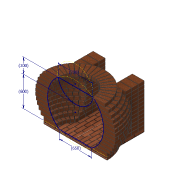
# Autodesk Inventor part: Geometria
Saved by Autodesk Inventor 2019.1 (Build 231200000, 200)
## iProperties
Created: 2019-11-21
Part Number: Geometria
Material: Brick, Common, Brown
Document SubType Name: Modeling
Designer: jjespitia
Density: 1.95 g/cm^3
Appearance: Uniform Running - Orange
Author: jjespitia
Autodesk Inventor part; units mm, degrees
ref_plane "YZ Plane" through (0, 0, 0) normal (1, 0, 0) x (0, 1, 0)
ref_plane "XZ Plane" through (0, 0, 0) normal (0, 1, 0) x (-1, 0, 0)
ref_plane "XY Plane" through (0, 0, 0) normal (0, 0, 1) x (1, 0, 0)
sketch "Sketch1" plane through (0, 0, 0) normal (0, 0, 1) x (1, 0, 0)
  circle A0 centre (0, 494.7917) radius 354.1667
  circle A1 centre (0, 0) radius 562.717
  line L0 (-325, -459.375) -> (325, -459.375)
  line L1 (-350, 440.625) -> (350, 440.625)
  line L2 (-350, 440.625) -> (0, 0)
  line L3 (0, 0) -> (0, 440.625)
  line L4 (0, -459.375) -> (0, 0)
  line L5 (0, 0) -> (-325, -459.375)
  dimension "d0" = 300
  dimension "d1" = 700
  dimension "d4" = 650
  dimension "d6" = 600
  dimension "d7" = 562.717
  dimension "d8" = 440.625
  dimension "d9" = 459.375
  constraints: 12 end point, 6 point on circle, 2 centre point, 2 horizontal, 2 midpoint, 1 coincident, 1 vertical
  measures "d0" distance edge to line of A0 L1
  measures "d1" distance of L1.start L1.end
  measures "d4" distance of L0.start L0.end
  measures "d6" distance edge to line of A0 L0
  measures "d7" distance of L1.start L2.end
  measures "d8" distance of L2.end L3.end
  measures "d9" distance of L4.start L2.end
sketch "Sketch2" plane through (0, 0, 0) normal (0, 0, 1) x (1, 0, 0)
  arc A0 (325, -459.375) -> (350, 440.625) centre (0, 0) ccw construction
  line L0 (562.3389, 20.625) -> (802.3389, 20.625)
  line L1 (802.3389, 20.625) -> (802.3389, -39.375)
  line L2 (802.3389, -39.375) -> (562.3389, -39.375)
  line L3 (562.3389, -39.375) -> (562.3389, 20.625)
  line L4 (560.5466, -49.375) -> (800.5466, -49.375)
  line L5 (800.5466, -49.375) -> (800.5466, -109.375)
  line L6 (800.5466, -109.375) -> (560.5466, -109.375)
  line L7 (560.5466, -109.375) -> (560.5466, -49.375)
  line L8 (549.9091, -119.375) -> (789.9091, -119.375)
  line L9 (789.9091, -119.375) -> (789.9091, -179.375)
  line L10 (789.9091, -179.375) -> (549.9091, -179.375)
  line L11 (549.9091, -179.375) -> (549.9091, -119.375)
  line L12 (350, 440.625) -> (590, 440.625)
  line L13 (590, 440.625) -> (590, 380.625)
  line L14 (590, 380.625) -> (350, 380.625)
  line L15 (350, 380.625) -> (350, 440.625)
  line L16 (423.4235, 370.625) -> (663.4235, 370.625)
  line L17 (663.4235, 370.625) -> (663.4235, 310.625)
  line L18 (663.4235, 310.625) -> (423.4235, 310.625)
  line L19 (423.4235, 310.625) -> (423.4235, 370.625)
  line L20 (475.6837, 300.625) -> (715.6837, 300.625)
  line L21 (715.6837, 300.625) -> (715.6837, 240.625)
  line L22 (715.6837, 240.625) -> (475.6837, 240.625)
  line L23 (475.6837, 240.625) -> (475.6837, 300.625)
  line L24 (513.286, 230.625) -> (753.286, 230.625)
  line L25 (753.286, 230.625) -> (753.286, 170.625)
  line L26 (753.286, 170.625) -> (513.286, 170.625)
  line L27 (513.286, 170.625) -> (513.286, 230.625)
  line L28 (539.3051, 160.625) -> (779.3051, 160.625)
  line L29 (779.3051, 160.625) -> (779.3051, 100.625)
  line L30 (779.3051, 100.625) -> (539.3051, 100.625)
  line L31 (539.3051, 100.625) -> (539.3051, 160.625)
  line L32 (555.3715, 90.625) -> (795.3715, 90.625)
  line L33 (795.3715, 90.625) -> (795.3715, 30.625)
  line L34 (795.3715, 30.625) -> (555.3715, 30.625)
  line L35 (555.3715, 30.625) -> (555.3715, 90.625)
  line L36 (529.8939, -189.375) -> (769.8939, -189.375)
  line L37 (769.8939, -189.375) -> (769.8939, -249.375)
  line L38 (769.8939, -249.375) -> (529.8939, -249.375)
  line L39 (529.8939, -249.375) -> (529.8939, -189.375)
  line L40 (499.3746, -259.375) -> (739.3746, -259.375)
  line L41 (739.3746, -259.375) -> (739.3746, -319.375)
  line L42 (739.3746, -319.375) -> (499.3746, -319.375)
  line L43 (499.3746, -319.375) -> (499.3746, -259.375)
  line L44 (456.2483, -329.375) -> (696.2483, -329.375)
  line L45 (696.2483, -329.375) -> (696.2483, -389.375)
  line L46 (696.2483, -389.375) -> (456.2483, -389.375)
  line L47 (456.2483, -389.375) -> (456.2483, -329.375)
  line L48 (396.4215, -399.375) -> (636.4215, -399.375)
  line L49 (636.4215, -399.375) -> (636.4215, -459.375)
  line L50 (636.4215, -459.375) -> (396.4215, -459.375)
  line L51 (396.4215, -459.375) -> (396.4215, -399.375)
  line L52 (0, -459.375) -> (636.4215, -459.375)
  line L53 (636.4215, -459.375) -> (636.4215, -519.375)
  line L54 (636.4215, -519.375) -> (0, -519.375)
  line L55 (0, -519.375) -> (0, -459.375)
  line L56 (0, -845.052) -> (0, 1131.2934) projected
  point P0 (0, 440.625)
  dimension "d10" = 60
  dimension "d11" = 240
  dimension "d15" = 60
  dimension "d16" = 240
  dimension "d17" = 60
  dimension "d18" = 240
  dimension "d19" = 10
  dimension "d20" = 10
  dimension "d21" = 60
  dimension "d22" = 240
  dimension "d23" = 60
  dimension "d24" = 240
  dimension "d25" = 60
  dimension "d26" = 240
  dimension "d27" = 10
  dimension "d28" = 10
  dimension "d29" = 60
  dimension "d30" = 240
  dimension "d31" = 60
  dimension "d32" = 240
  dimension "d33" = 60
  dimension "d34" = 240
  dimension "d35" = 10
  dimension "d36" = 10
  dimension "d37" = 10
  dimension "d38" = 10
  dimension "d39" = 60
  dimension "d40" = 240
  dimension "d41" = 60
  dimension "d42" = 240
  dimension "d43" = 60
  dimension "d44" = 240
  dimension "d45" = 10
  dimension "d46" = 10
  dimension "d47" = 60
  dimension "d48" = 240
  dimension "d55" = 10
  dimension "d56" = 10
  constraints: 112 end point, 28 parallel, 14 horizontal, 14 perpendicular, 2 coincident, 1 collinear, 1 point on line, 16 other
  measures "d10" distance of L0.end L1.end
  measures "d11" distance of L0.start L0.end
  measures "d15" distance of L4.end L5.end
  measures "d16" distance of L4.start L4.end
  measures "d17" distance of L8.end L9.end
  measures "d18" distance of L8.start L8.end
  measures "d19" distance between parallel lines of L4 L2
  measures "d20" distance between parallel lines of L8 L6
  measures "d21" distance of L13.start L13.end
  measures "d22" distance of L12.start L13.start
  measures "d23" distance of L16.end L18.start
  measures "d24" distance of L16.start L16.end
  measures "d25" distance of L20.end L21.end
  measures "d26" distance of L23.end L20.end
  measures "d27" distance between parallel lines of L16 L14
  measures "d28" distance between parallel lines of L20 L18
  measures "d29" distance of L25.start L25.end
  measures "d30" distance of L24.start L25.start
  measures "d31" distance of L28.end L30.start
  measures "d32" distance of L28.start L28.end
  measures "d33" distance of L32.end L33.end
  measures "d34" distance of L35.end L32.end
  measures "d35" distance between parallel lines of L28 L26
  measures "d36" distance between parallel lines of L32 L30
  measures "d37" distance between parallel lines of L22 L24
  measures "d38" distance between parallel lines of L34 L0
  measures "d39" distance of L37.start L37.end
  measures "d40" distance of L36.start L37.start
  measures "d41" distance of L40.end L42.start
  measures "d42" distance of L40.start L40.end
  measures "d43" distance of L44.end L45.end
  measures "d44" distance of L47.end L44.end
  measures "d45" distance between parallel lines of L40 L38
  measures "d46" distance between parallel lines of L44 L42
  measures "d47" distance of L49.start L49.end
  measures "d48" distance of L48.start L49.start
  measures "d55" distance between parallel lines of L10 L36
  measures "d56" distance between parallel lines of L48 L46
revolve "Revolution1" add sketch "Sketch2" angle 180 about axis through (0, -10, 0) along (0, 1, 0) contours L0 L1 L2 L3 | L8 L9 L10 L11 | L12 L13 L14 L15 | L20 L21 L22 L23 | L28 L29 L30 L31 | L40 L41 L42 L43 | L48 L49 L50 L51
revolve "Revolution2" add sketch "Sketch2" angle 180 about axis through (0, -10, 0) along (0, 1, 0) separate body contours L4 L5 L6 L7 | L16 L17 L18 L19 | L24 L25 L26 L27 | L32 L33 L34 L35 | L36 L37 L38 L39 | L44 L45 L46 L47 | L50 L53 L54 L55 L52
sketch "Sketch3" plane through (350, 440.625, 0) normal (0, 0, 1) x (1, 0, 0)
  line L0 (-625, -70) -> (-75, -70)
  line L1 (-75, -70) -> (-75, -900)
  line L2 (-75, -900) -> (-625, -900)
  line L3 (-625, -900) -> (-625, -70)
  line L4 (73.4235, -70) -> (-773.4235, -70) projected
  line L5 (286.4215, -900) -> (-986.4215, -900) projected
  point P0 (-350, -440.625)
  point P1 (-350, -70)
  dimension "d60" = 550
  constraints: 8 end point, 2 parallel, 2 point on line, 1 horizontal, 1 midpoint, 1 perpendicular, 1 vertical alignment
  measures "d60" distance of L1.end L2.end
extrude "Extrusion1" cut sketch "Sketch3" against normal through all bodies 2 1
sketch "Sketch4" plane through (0, -459.375, 0) normal (0, 1, 0) x (1, 0, 0)
  line L0 (275, 490.5099) -> (-275, 490.5099) construction
  line L1 (515, 490.5099) -> (275, 490.5099)
  line L2 (275, 490.5099) -> (275, 610.5099)
  line L3 (275, 610.5099) -> (515, 610.5099)
  line L4 (515, 610.5099) -> (515, 490.5099)
  line L5 (-275, 490.5099) -> (-515, 490.5099)
  line L6 (-515, 490.5099) -> (-515, 610.5099)
  line L7 (-515, 610.5099) -> (-275, 610.5099)
  line L8 (-275, 610.5099) -> (-275, 490.5099)
  line L9 (515, 620.5099) -> (275, 620.5099)
  line L10 (275, 620.5099) -> (275, 740.5099)
  line L11 (275, 740.5099) -> (515, 740.5099)
  line L12 (515, 740.5099) -> (515, 620.5099)
  line L13 (-275, 620.5099) -> (-515, 620.5099)
  line L14 (-515, 620.5099) -> (-515, 740.5099)
  line L15 (-515, 740.5099) -> (-275, 740.5099)
  line L16 (-275, 740.5099) -> (-275, 620.5099)
  line L17 (515, 870.5099) -> (275, 870.5099)
  line L18 (275, 870.5099) -> (275, 750.5099)
  line L19 (275, 750.5099) -> (515, 750.5099)
  line L20 (515, 750.5099) -> (515, 870.5099)
  line L21 (-275, 870.5099) -> (-515, 870.5099)
  line L22 (-515, 870.5099) -> (-515, 750.5099)
  line L23 (-515, 750.5099) -> (-275, 750.5099)
  line L24 (-275, 750.5099) -> (-275, 870.5099)
  point P0 (0, 0)
  point P1 (-275, 490.5099)
  dimension "d63" = 120
  dimension "d64" = 240
  dimension "d65" = 10
  dimension "d66" = 10
  dimension "d67" = 10
  dimension "d68" = 10
  constraints: 51 end point, 12 parallel, 10 equal length, 7 horizontal, 6 perpendicular, 4 collinear, 1 coincident
  measures "d63" distance between parallel lines of L3 L1
  measures "d64" distance between parallel lines of L4 L2
  measures "d65" distance between parallel lines of L3 L9
  measures "d66" distance between parallel lines of L7 L13
  measures "d67" distance between parallel lines of L19 L11
  measures "d68" distance between parallel lines of L23 L15
extrude "Extrusion2" add sketch "Sketch4" along normal up to surface (830 mm away) separate body
sketch "Sketch5" plane through (636.4215, -519.375, 0) normal (0, 0, 1) x (1, 0, 0)
  line L0 (-1438.7604, 830) -> (165.9174, 830)
  line L1 (165.9174, 830) -> (165.9174, 820)
  line L2 (165.9174, 820) -> (-1438.7604, 820)
  line L3 (-1438.7604, 820) -> (-1438.7604, 830)
  line L4 (-1438.7604, 540) -> (-1438.7604, 480) projected
  line L5 (165.9174, 540) -> (165.9174, 480) projected
  line L6 (-1438.7604, 760) -> (165.9174, 760)
  line L7 (165.9174, 760) -> (165.9174, 750)
  line L8 (165.9174, 750) -> (-1438.7604, 750)
  line L9 (-1438.7604, 750) -> (-1438.7604, 760)
  line L10 (-1438.7604, 690) -> (165.9174, 690)
  line L11 (165.9174, 690) -> (165.9174, 680)
  line L12 (165.9174, 680) -> (-1438.7604, 680)
  line L13 (-1438.7604, 680) -> (-1438.7604, 690)
  line L14 (-1438.7604, 620) -> (165.9174, 620)
  line L15 (165.9174, 620) -> (165.9174, 610)
  line L16 (165.9174, 610) -> (-1438.7604, 610)
  line L17 (-1438.7604, 610) -> (-1438.7604, 620)
  line L18 (-1438.7604, 550) -> (165.9174, 550)
  line L19 (165.9174, 550) -> (165.9174, 540)
  line L20 (165.9174, 540) -> (-1438.7604, 540)
  line L21 (-1438.7604, 540) -> (-1438.7604, 550)
  line L22 (-1438.7604, 480) -> (165.9174, 480)
  line L23 (165.9174, 480) -> (165.9174, 470)
  line L24 (165.9174, 470) -> (-1438.7604, 470)
  line L25 (-1438.7604, 470) -> (-1438.7604, 480)
  line L26 (-1438.7604, 410) -> (165.9174, 410)
  line L27 (165.9174, 410) -> (165.9174, 400)
  line L28 (165.9174, 400) -> (-1438.7604, 400)
  line L29 (-1438.7604, 400) -> (-1438.7604, 410)
  line L30 (-1438.7604, 340) -> (165.9174, 340)
  line L31 (165.9174, 340) -> (165.9174, 330)
  line L32 (165.9174, 330) -> (-1438.7604, 330)
  line L33 (-1438.7604, 330) -> (-1438.7604, 340)
  line L34 (-1438.7604, 270) -> (165.9174, 270)
  line L35 (165.9174, 270) -> (165.9174, 260)
  line L36 (165.9174, 260) -> (-1438.7604, 260)
  line L37 (-1438.7604, 260) -> (-1438.7604, 270)
  line L38 (-1438.7604, 200) -> (165.9174, 200)
  line L39 (165.9174, 200) -> (165.9174, 190)
  line L40 (165.9174, 190) -> (-1438.7604, 190)
  line L41 (-1438.7604, 190) -> (-1438.7604, 200)
  line L42 (-1438.7604, 130) -> (165.9174, 130)
  line L43 (165.9174, 130) -> (165.9174, 120)
  line L44 (165.9174, 120) -> (-1438.7604, 120)
  line L45 (-1438.7604, 120) -> (-1438.7604, 130)
  point P0 (-636.4215, 519.375)
  point P1 (27.0021, 830)
  point P2 (79.2622, 820)
  point P3 (27.0021, 760)
  point P4 (79.2622, 750)
  point P5 (27.0021, 690)
  point P6 (79.2622, 680)
  point P7 (27.0021, 620)
  point P8 (79.2622, 610)
  point P9 (27.0021, 550)
  point P10 (79.2622, 540)
  point P11 (27.0021, 480)
  point P12 (79.2622, 470)
  point P13 (27.0021, 410)
  point P14 (79.2622, 400)
  point P15 (27.0021, 340)
  point P16 (79.2622, 330)
  point P17 (27.0021, 270)
  point P18 (79.2622, 260)
  point P19 (27.0021, 200)
  point P20 (79.2622, 190)
  point P21 (27.0021, 130)
  point P22 (79.2622, 120)
  dimension "d73" = 70
  constraints: 88 end point, 22 point on line, 3 collinear, 2 parallel, 1 horizontal, 1 perpendicular, 1 vertical, 99 other
  measures "d73" distance of L0.start L6.start
extrude "Extrusion3" cut sketch "Sketch5" against normal up to surface (870.5099 mm away) contours L0 L1 L2 L3 | L21 L18 L19 L20 | L22 L23 L24 L25 | L6 L7 L8 L9 | L10 L11 L12 L13 | L14 L15 L16 L17 | L26 L27 L28 L29 | L30 L31 L32 L33 | L34 L35 L36 L37 | L38 L39 L40 L41 | L42 L43 L44 L45 bodies 3
sketch "Sketch6" plane through (350, 440.625, 0) normal (0, 1, 0) x (1, 0, 0)
  arc A0 (0, 0) -> (-700, 0) centre (-350, 0) ccw projected
  line L0 (-350.7786, 4.939) -> (-349.2214, -4.939)
  line L1 (-349.2214, -4.939) -> (572.3389, 140.34)
  line L2 (572.3389, 140.34) -> (570.7817, 150.218)
  line L3 (570.7817, 150.218) -> (-350.7786, 4.939)
  arc A1 (452.3389, 0) -> (-75, 753.7391) centre (-350, 0) ccw construction
  line L4 (-351.5026, 4.7689) -> (-348.4974, -4.7689)
  line L5 (-348.4974, -4.7689) -> (541.3175, 275.6038)
  line L6 (541.3175, 275.6038) -> (538.3122, 285.1415)
  line L7 (538.3122, 285.1415) -> (-351.5026, 4.7689)
  line L8 (-352.1934, 4.4932) -> (-347.8066, -4.4932)
  line L9 (-347.8066, -4.4932) -> (490.5748, 404.7695)
  line L10 (490.5748, 404.7695) -> (486.188, 413.756)
  line L11 (486.188, 413.756) -> (-352.1934, 4.4932)
  line L12 (-352.8356, 4.1181) -> (-347.1644, -4.1181)
  line L13 (-347.1644, -4.1181) -> (421.2334, 524.9793)
  line L14 (421.2334, 524.9793) -> (415.5621, 533.2156)
  line L15 (415.5621, 533.2156) -> (-352.8356, 4.1181)
  line L16 (-353.4151, 3.652) -> (-346.5849, -3.652)
  line L17 (-346.5849, -3.652) -> (334.8278, 633.5734)
  line L18 (334.8278, 633.5734) -> (327.9975, 640.8773)
  line L19 (327.9975, 640.8773) -> (-353.4151, 3.652)
  line L20 (-353.9191, 3.105) -> (-346.0809, -3.105)
  line L21 (-346.0809, -3.105) -> (233.2695, 728.149)
  line L22 (233.2695, 728.149) -> (225.4314, 734.3589)
  line L23 (225.4314, 734.3589) -> (-353.9191, 3.105)
  line L24 (-354.3363, 2.4893) -> (-345.6637, -2.4893)
  line L25 (-345.6637, -2.4893) -> (118.8059, 806.6135)
  line L26 (118.8059, 806.6135) -> (110.1333, 811.5921)
  line L27 (110.1333, 811.5921) -> (-354.3363, 2.4893)
  line L28 (-354.6576, 1.8185) -> (-345.3424, -1.8185)
  line L29 (-345.3424, -1.8185) -> (-6.0306, 867.2309)
  line L30 (-6.0306, 867.2309) -> (-15.3458, 870.8679)
  line L31 (-15.3458, 870.8679) -> (-354.6576, 1.8185)
  line L32 (-354.8758, 1.1075) -> (-345.1242, -1.1075)
  line L33 (-345.1242, -1.1075) -> (-138.4778, 908.6598)
  line L34 (-138.4778, 908.6598) -> (-148.2294, 910.8748)
  line L35 (-148.2294, 910.8748) -> (-354.8758, 1.1075)
  line L36 (-354.9861, 0.372) -> (-345.0139, -0.372)
  line L37 (-345.0139, -0.372) -> (-275.6051, 929.9837)
  line L38 (-275.6051, 929.9837) -> (-285.5774, 930.7277)
  line L39 (-285.5774, 930.7277) -> (-354.9861, 0.372)
  line L40 (-354.9862, -0.3718) -> (-345.0138, 0.3718)
  line L41 (-345.0138, 0.3718) -> (-414.3785, 930.7307)
  line L42 (-414.3785, 930.7307) -> (-424.3509, 929.9872)
  line L43 (-424.3509, 929.9872) -> (-354.9862, -0.3718)
  line L44 (-354.8759, -1.1073) -> (-345.1241, 1.1073)
  line L45 (-345.1241, 1.1073) -> (-551.7275, 910.8844)
  line L46 (-551.7275, 910.8844) -> (-561.4792, 908.6698)
  line L47 (-561.4792, 908.6698) -> (-354.8759, -1.1073)
  line L48 (-354.6577, -1.8183) -> (-345.3423, 1.8183)
  line L49 (-345.3423, 1.8183) -> (-684.613, 870.8837)
  line L50 (-684.613, 870.8837) -> (-693.9283, 867.2471)
  line L51 (-693.9283, 867.2471) -> (-354.6577, -1.8183)
  line L52 (-354.3364, -2.4891) -> (-345.6636, 2.4891)
  line L53 (-345.6636, 2.4891) -> (-810.0949, 811.6138)
  line L54 (-810.0949, 811.6138) -> (-818.7677, 806.6357)
  line L55 (-818.7677, 806.6357) -> (-354.3364, -2.4891)
  line L56 (-353.9192, -3.1048) -> (-346.0808, 3.1048)
  line L57 (-346.0808, 3.1048) -> (-925.3966, 734.3861)
  line L58 (-925.3966, 734.3861) -> (-933.2351, 728.1766)
  line L59 (-933.2351, 728.1766) -> (-353.9192, -3.1048)
  line L60 (-353.4153, -3.6518) -> (-346.5847, 3.6518)
  line L61 (-346.5847, 3.6518) -> (-1027.9671, 640.9094)
  line L62 (-1027.9671, 640.9094) -> (-1034.7978, 633.6058)
  line L63 (-1034.7978, 633.6058) -> (-353.4153, -3.6518)
  line L64 (-352.8358, -4.118) -> (-347.1642, 4.118)
  line L65 (-347.1642, 4.118) -> (-1115.5369, 533.2518)
  line L66 (-1115.5369, 533.2518) -> (-1121.2086, 525.0158)
  line L67 (-1121.2086, 525.0158) -> (-352.8358, -4.118)
  line L68 (-352.1936, -4.4931) -> (-347.8064, 4.4931)
  line L69 (-347.8064, 4.4931) -> (-1186.1684, 413.7955)
  line L70 (-1186.1684, 413.7955) -> (-1190.5556, 404.8093)
  line L71 (-1190.5556, 404.8093) -> (-352.1936, -4.4931)
  line L72 (-351.5029, -4.7688) -> (-348.4971, 4.7688)
  line L73 (-348.4971, 4.7688) -> (-1238.2987, 285.1836)
  line L74 (-1238.2987, 285.1836) -> (-1241.3044, 275.646)
  line L75 (-1241.3044, 275.646) -> (-351.5029, -4.7688)
  line L76 (-350.7788, -4.939) -> (-349.2212, 4.939)
  line L77 (-349.2212, 4.939) -> (-1270.7745, 150.2616)
  line L78 (-1270.7745, 150.2616) -> (-1272.3322, 140.3837)
  line L79 (-1272.3322, 140.3837) -> (-350.7788, -4.939)
  line L80 (429.3051, 0) -> (189.3051, 0) projected
  point P0 (-350, 0)
  point P1 (-350, 0)
  point P2 (443.3143, 120)
  point P3 (-350, 0)
  point P4 (-3.8721, 51.9177)
  point P5 (-350, 0)
  point P6 (416.7375, 236.3498)
  point P7 (443.4626, 119.016)
  point P8 (-350, 0)
  point P9 (-15.4026, 102.6867)
  point P10 (-350, 0)
  point P11 (373.1958, 347.4701)
  point P12 (417.0301, 235.3986)
  point P13 (-350, 0)
  point P14 (-34.3364, 151.1836)
  point P15 (-350, 0)
  point P16 (313.6527, 450.9022)
  point P17 (373.6262, 346.5728)
  point P18 (-350, 0)
  point P19 (-60.2546, 196.3354)
  point P20 (-350, 0)
  point P21 (239.4255, 544.3576)
  point P22 (314.2114, 450.0787)
  point P23 (-350, 0)
  point P24 (-92.5837, 237.1432)
  point P25 (-350, 0)
  point P26 (152.1566, 625.7686)
  point P27 (240.1002, 543.6262)
  point P28 (-350, 0)
  point P29 (-130.6085, 272.7038)
  point P30 (-350, 0)
  point P31 (53.7771, 693.3338)
  point P32 (152.9324, 625.1453)
  point P33 (-350, 0)
  point P34 (-173.4875, 302.2306)
  point P35 (-350, 0)
  point P36 (-53.5365, 745.5582)
  point P37 (54.6367, 692.8325)
  point P38 (-350, 0)
  point P39 (-220.272, 325.0702)
  point P40 (-350, 0)
  point P41 (-167.4097, 781.2864)
  point P42 (-52.6121, 745.19)
  point P43 (-350, 0)
  point P44 (-269.927, 340.7173)
  point P45 (-350, 0)
  point P46 (-285.3228, 799.7278)
  point P47 (-166.4408, 781.0593)
  point P48 (-350, 0)
  point P49 (-321.3536, 348.8257)
  point P50 (-350, 0)
  point P51 (-404.667, 800.4743)
  point P52 (-284.331, 799.6469)
  point P53 (-350, 0)
  point P54 (-373.414, 349.216)
  point P55 (-350, 0)
  point P56 (-522.8017, 783.5096)
  point P57 (-403.6742, 800.5415)
  point P58 (-350, 0)
  point P59 (-424.9564, 341.8794)
  point P60 (-350, 0)
  point P61 (-637.1129, 749.2088)
  point P62 (-521.8298, 783.7233)
  point P63 (-350, 0)
  point P64 (-474.8403, 326.9784)
  point P65 (-350, 0)
  point P66 (-745.0714, 698.331)
  point P67 (-636.1834, 749.5643)
  point P68 (-350, 0)
  point P69 (-521.9619, 304.8427)
  point P70 (-350, 0)
  point P71 (-844.2886, 632.0019)
  point P72 (-744.205, 698.8205)
  point P73 (-350, 0)
  point P74 (-565.2788, 275.962)
  point P75 (-350, 0)
  point P76 (-932.5691, 551.6891)
  point P77 (-843.5044, 632.6145)
  point P78 (-350, 0)
  point P79 (-603.8323, 240.9754)
  point P80 (-350, 0)
  point P81 (-1007.9597, 459.1696)
  point P82 (-931.8844, 552.4112)
  point P83 (-350, 0)
  point P84 (-636.7696, 200.6569)
  point P85 (-350, 0)
  point P86 (-1068.7922, 356.4905)
  point P87 (-1007.3897, 459.9853)
  point P88 (-350, 0)
  point P89 (-663.3618, 155.8987)
  point P90 (-350, 0)
  point P91 (-1113.7206, 245.9236)
  point P92 (-1068.3495, 357.3817)
  point P93 (-350, 0)
  point P94 (-683.0205, 107.6911)
  point P95 (-350, 0)
  point P96 (-1141.751, 129.9155)
  point P97 (-1113.415, 246.8707)
  dimension "d82" = 10
  dimension "d83" = 120
  dimension "d84" = 120
  dimension "d87" = 162.08
  dimension "d89" = 8.959
  constraints: 160 end point, 21 coincident, 20 point on line, 2 parallel, 1 midpoint, 1 perpendicular, 1 point on circle, 285 other
  measures "d82" distance between parallel lines of L1 L3
  measures "d83" vertical distance of A1.start point (443.314, 120)
  measures "d84" horizontal distance of L1.end A1.start
  measures "d89" angle of L80 L1
extrude "Extrusion4" cut sketch "Sketch6" against normal up to surface (900 mm away) contours L1 L0 L4 L5 L3 A0 | A0 L3 L2 L1 | L5 L3 L9 L7 A0 | A0 L7 L6 L5 | L5 L4 L8 L9 L3 | L4 L7 L77 L3 L0 | L8 L11 L77 L7 L4 | L12 L15 L77 L11 L8 | L12 L13 L3 L9 L8 | L16 L19 L77 L15 L12 | L16 L17 L3 L13 L12 | L20 L23 L77 L19 L16 | L20 L21 L3 L17 L16 | L24 L27 L77 L23 L20 | L24 L25 L3 L21 L20 | L28 L31 L77 L27 L24 | L28 L29 L3 L25 L24 | L32 L35 L77 L31 L28 | L32 L33 L3 L29 L28 | L36 L39 L77 L35 L32 | L36 L37 L3 L33 L32 | L40 L43 L77 L39 L36 | L40 L41 L3 L37 L36 | L44 L47 L77 L43 L40 | L44 L45 L3 L41 L40 | L48 L51 L77 L47 L44 | L48 L49 L3 L45 L44 | L52 L55 L77 L51 L48 | L52 L53 L3 L49 L48 | L56 L59 L77 L55 L52 | L56 L57 L3 L53 L52 | L60 L63 L77 L59 L56 | L60 L61 L3 L57 L56 | L64 L67 L77 L63 L60 | L64 L65 L3 L61 L60 | L68 L71 L77 L67 L64 | L68 L69 L3 L65 L64 | L72 L75 L77 L71 L68 | L72 L73 L3 L69 L68 | L76 L79 A0 L77 L75 L72 | L76 L77 L3 L73 L72 | L0 L3 L77 L76 | L3 L13 L7 L9 | L9 L7 L13 L11 A0 | A0 L11 L10 L9 | L3 L17 L7 L13 | L77 L7 L73 L3 | L77 L11 L73 L7 | L77 L15 L73 L11 | L77 L19 L73 L15 | L77 L23 L73 L19 | L3 L21 L7 L17 | L77 L27 L73 L23 | L3 L25 L7 L21 | L77 L31 L73 L27 | L3 L29 L7 L25 | L77 L35 L73 L31 | L3 L33 L7 L29 | L77 L39 L73 L35 | L3 L37 L7 L33 | L77 L43 L73 L39 | L3 L41 L7 L37 | L77 L47 L73 L43 | L3 L45 L7 L41 | L77 L51 L73 L47 | L3 L49 L7 L45 | L77 L55 L73 L51 | L3 L53 L7 L49 | L77 L59 L73 L55 | L3 L57 L7 L53 | L77 L63 L73 L59 | L3 L61 L7 L57 | L77 L67 L73 L63 | L3 L65 L7 L61 | L77 L71 L73 L67 | L3 L69 L7 L65 | L77 L75 A0 L73 L71 | L3 L73 L7 L69 | L79 L78 L77 A0 | L7 L17 L11 L13 | L73 L11 L69 L7 | L73 L15 L69 L11 | L73 L19 L69 L15 | L73 L23 L69 L19 | L7 L21 L11 L17 | L73 L27 L69 L23 | L7 L25 L11 L21 | L73 L31 L69 L27 | L7 L29 L11 L25 | L73 L35 L69 L31 | L7 L33 L11 L29 | L73 L39 L69 L35 | L7 L37 L11 L33 | L73 L43 L69 L39 | L7 L41 L11 L37 | L73 L47 L69 L43 | L7 L45 L11 L41 | L73 L51 L69 L47 | L7 L49 L11 L45 | L73 L55 L69 L51 | L7 L53 L11 L49 | L73 L59 L69 L55 | L7 L57 L11 L53 | L73 L63 L69 L59 | L7 L61 L11 L57 | L73 L67 L69 L63 | L7 L65 L11 L61 | L73 L71 A0 L69 L67 | L7 L69 L11 L65 | L75 L74 L73 A0 | L13 L11 L17 L15 A0 | A0 L15 L14 L13 | L69 L15 L65 L11 | L69 L19 L65 L15 | L69 L23 L65 L19 | L11 L21 L15 L17 | L69 L27 L65 L23 | L11 L25 L15 L21 | L69 L31 L65 L27 | L11 L29 L15 L25 | L69 L35 L65 L31 | L11 L33 L15 L29 | L69 L39 L65 L35 | L11 L37 L15 L33 | L69 L43 L65 L39 | L11 L41 L15 L37 | L69 L47 L65 L43 | L11 L45 L15 L41 | L69 L51 L65 L47 | L11 L49 L15 L45 | L69 L55 L65 L51 | L11 L53 L15 L49 | L69 L59 L65 L55 | L11 L57 L15 L53 | L69 L63 L65 L59 | L11 L61 L15 L57 | L69 L67 A0 L65 L63 | L11 L65 L15 L61 | L71 L70 L69 A0 | L65 L19 L61 L15 | L65 L23 L61 L19 | L15 L21 L19 A0 L17 | L65 L27 L61 L23 | L15 L25 L19 L21 | L65 L31 L61 L27 | L15 L29 L19 L25 | L65 L35 L61 L31 | L15 L33 L19 L29 | L65 L39 L61 L35 | L15 L37 L19 L33 | L65 L43 L61 L39 | L15 L41 L19 L37 | L65 L47 L61 L43 | L15 L45 L19 L41 | L65 L51 L61 L47 | L15 L49 L19 L45 | L65 L55 L61 L51 | L15 L53 L19 L49 | L65 L59 L61 L55 | L15 L57 L19 L53 | L65 L63 A0 L61 L59 | L15 L61 L19 L57 | L67 L66 L65 A0 | A0 L19 L18 L17 | L61 L23 L57 L19 | L61 L27 L57 L23 | L19 L25 L23 A0 L21 | L61 L31 L57 L27 | L19 L29 L23 L25 | L61 L35 L57 L31 | L19 L33 L23 L29 | L61 L39 L57 L35 | L19 L37 L23 L33 | L61 L43 L57 L39 | L19 L41 L23 L37 | L61 L47 L57 L43 | L19 L45 L23 L41 | L61 L51 L57 L47 | L19 L49 L23 L45 | L61 L55 L57 L51 | L19 L53 L23 L49 | L61 L59 A0 L57 L55 | L19 L57 L23 L53 | L63 L62 L61 A0 | L57 L27 L53 L23 | A0 L23 L22 L21 | L57 L31 L53 L27 | L23 L29 L27 A0 L25 | L57 L35 L53 L31 | L23 L33 L27 L29 | L57 L39 L53 L35 | L23 L37 L27 L33 | L57 L43 L53 L39 | L23 L41 L27 L37 | L57 L47 L53 L43 | L23 L45 L27 L41 | L57 L51 L53 L47 | L23 L49 L27 L45 | L57 L55 A0 L53 L51 | L23 L53 L27 L49 | L59 L58 L57 A0 | L53 L31 L49 L27 | A0 L27 L26 L25 | L53 L35 L49 L31 | L27 L33 L31 A0 L29 | L53 L39 L49 L35 | L27 L37 L31 L33 | L53 L43 L49 L39 | L27 L41 L31 L37 | L53 L47 L49 L43 | L27 L45 L31 L41 | L53 L51 A0 L49 L47 | L27 L49 L31 L45 | L55 L54 L53 A0 | L49 L35 L45 L31 | A0 L31 L30 L29 | L49 L39 L45 L35 | L31 L37 L35 A0 L33 | L49 L43 L45 L39 | L31 L41 L35 L37 | L49 L47 A0 L45 L43 | L31 L45 L35 L41 | L51 L50 L49 A0 | L45 L39 L41 L35 | A0 L35 L34 L33 | L45 L43 A0 L41 L39 | L35 L41 L39 A0 L37 | L47 L46 L45 A0 | A0 L39 L38 L37 | L43 L42 L41 A0 bodies 1
sketch "Sketch7" plane through (-663.4235, 370.625, 0) normal (0, 1, 0) x (1, 0, 0)
  line L0 (663.8606, -4.9809) -> (1609.6391, 78.015)
  line L1 (1609.6391, 78.015) -> (1608.7649, 87.9767)
  line L2 (1608.7649, 87.9767) -> (662.9865, 4.9809)
  line L3 (662.9865, 4.9809) -> (663.8606, -4.9809)
  arc A0 (1463.9702, 0) -> (938.4235, 751.831) centre (663.4235, 0) ccw construction
  line L4 (1326.8471, 0) -> (1086.8471, 0) projected
  arc A1 (1086.8471, 0) -> (938.4235, 321.9666) centre (663.4235, 0) ccw projected
  line L5 (664.6298, -4.8523) -> (1586, 224.1939)
  line L6 (1586, 224.1939) -> (1583.5875, 233.8986)
  line L7 (1583.5875, 233.8986) -> (662.2173, 4.8523)
  line L8 (662.2173, 4.8523) -> (664.6298, -4.8523)
  line L9 (665.3696, -4.6057) -> (1539.9189, 364.9193)
  line L10 (1539.9189, 364.9193) -> (1536.0268, 374.1308)
  line L11 (1536.0268, 374.1308) -> (661.4775, 4.6057)
  line L12 (661.4775, 4.6057) -> (665.3696, -4.6057)
  line L13 (666.0621, -4.2471) -> (1472.5168, 496.7679)
  line L14 (1472.5168, 496.7679) -> (1467.2397, 505.2622)
  line L15 (1467.2397, 505.2622) -> (660.785, 4.2471)
  line L16 (660.785, 4.2471) -> (666.0621, -4.2471)
  line L17 (666.6904, -3.7852) -> (1385.4332, 616.5325)
  line L18 (1385.4332, 616.5325) -> (1378.8995, 624.1029)
  line L19 (1378.8995, 624.1029) -> (660.1567, 3.7852)
  line L20 (660.1567, 3.7852) -> (666.6904, -3.7852)
  line L21 (667.2392, -3.2312) -> (1280.7865, 721.2997)
  line L22 (1280.7865, 721.2997) -> (1273.1552, 727.762)
  line L23 (1273.1552, 727.762) -> (659.6079, 3.2312)
  line L24 (659.6079, 3.2312) -> (667.2392, -3.2312)
  line L25 (667.6952, -2.5986) -> (1161.1223, 808.521)
  line L26 (1161.1223, 808.521) -> (1152.5789, 813.7182)
  line L27 (1152.5789, 813.7182) -> (659.1519, 2.5986)
  line L28 (659.1519, 2.5986) -> (667.6952, -2.5986)
  line L29 (668.0473, -1.9028) -> (1029.3513, 876.0748)
  line L30 (1029.3513, 876.0748) -> (1020.1038, 879.8804)
  line L31 (1020.1038, 879.8804) -> (658.7998, 1.9028)
  line L32 (658.7998, 1.9028) -> (668.0473, -1.9028)
  line L33 (668.287, -1.1607) -> (888.6791, 922.3178)
  line L34 (888.6791, 922.3178) -> (878.9523, 924.6392)
  line L35 (878.9523, 924.6392) -> (658.5601, 1.1607)
  line L36 (658.5601, 1.1607) -> (668.287, -1.1607)
  line L37 (668.4083, -0.3903) -> (742.5274, 946.1252)
  line L38 (742.5274, 946.1252) -> (732.558, 946.9058)
  line L39 (732.558, 946.9058) -> (658.4388, 0.3903)
  line L40 (658.4388, 0.3903) -> (668.4083, -0.3903)
  line L41 (668.4084, 0.3895) -> (594.4515, 946.9177)
  line L42 (594.4515, 946.9177) -> (584.4819, 946.1387)
  line L43 (584.4819, 946.1387) -> (658.4387, -0.3895)
  line L44 (658.4387, -0.3895) -> (668.4084, 0.3895)
  line L45 (668.2872, 1.1598) -> (448.0534, 924.6761)
  line L46 (448.0534, 924.6761) -> (438.3262, 922.3565)
  line L47 (438.3262, 922.3565) -> (658.5599, -1.1598)
  line L48 (658.5599, -1.1598) -> (668.2872, 1.1598)
  line L49 (668.0477, 1.902) -> (306.8942, 879.9415)
  line L50 (306.8942, 879.9415) -> (297.646, 876.1376)
  line L51 (297.646, 876.1376) -> (658.7994, -1.902)
  line L52 (658.7994, -1.902) -> (668.0477, 1.902)
  line L53 (667.6957, 2.5979) -> (174.4078, 813.8021)
  line L54 (174.4078, 813.8021) -> (165.8635, 808.6064)
  line L55 (165.8635, 808.6064) -> (659.1514, -2.5979)
  line L56 (659.1514, -2.5979) -> (667.6957, 2.5979)
  line L57 (667.2398, 3.2305) -> (53.8167, 727.8666)
  line L58 (53.8167, 727.8666) -> (46.1843, 721.4055)
  line L59 (46.1843, 721.4055) -> (659.6073, -3.2305)
  line L60 (659.6073, -3.2305) -> (667.2398, 3.2305)
  line L61 (666.691, 3.7846) -> (-51.9454, 624.2256)
  line L62 (-51.9454, 624.2256) -> (-58.4804, 616.6563)
  line L63 (-58.4804, 616.6563) -> (660.156, -3.7846)
  line L64 (660.156, -3.7846) -> (666.691, 3.7846)
  line L65 (666.0628, 4.2467) -> (-140.3059, 505.4)
  line L66 (-140.3059, 505.4) -> (-145.5845, 496.9067)
  line L67 (-145.5845, 496.9067) -> (660.7843, -4.2467)
  line L68 (660.7843, -4.2467) -> (666.0628, 4.2467)
  line L69 (665.3704, 4.6054) -> (-209.1155, 374.2804)
  line L70 (-209.1155, 374.2804) -> (-213.0092, 365.0696)
  line L71 (-213.0092, 365.0696) -> (661.4767, -4.6054)
  line L72 (661.4767, -4.6054) -> (665.3704, 4.6054)
  line L73 (664.6306, 4.8521) -> (-256.7003, 234.0564)
  line L74 (-256.7003, 234.0564) -> (-259.1145, 224.3522)
  line L75 (-259.1145, 224.3522) -> (662.2165, -4.8521)
  line L76 (662.2165, -4.8521) -> (664.6306, 4.8521)
  line L77 (663.8615, 4.9808) -> (-281.9027, 88.1388)
  line L78 (-281.9027, 88.1388) -> (-282.7786, 78.1773)
  line L79 (-282.7786, 78.1773) -> (662.9856, -4.9808)
  line L80 (662.9856, -4.9808) -> (663.8615, 4.9808)
  point P0 (663.4235, 0)
  point P1 (663.4235, 0)
  point P2 (1461.327, 65)
  point P3 (663.4235, 0)
  point P4 (1441.5154, 188.2761)
  point P5 (663.4235, 0)
  point P6 (663.4235, 0)
  point P7 (1402.7766, 306.9723)
  point P8 (663.4235, 0)
  point P9 (663.4235, 0)
  point P10 (1346.0527, 418.2013)
  point P11 (663.4235, 0)
  point P12 (663.4235, 0)
  point P13 (1272.7236, 519.2574)
  point P14 (663.4235, 0)
  point P15 (663.4235, 0)
  point P16 (1184.5732, 607.6824)
  point P17 (663.4235, 0)
  point P18 (663.4235, 0)
  point P19 (1083.7456, 681.3254)
  point P20 (663.4235, 0)
  point P21 (663.4235, 0)
  point P22 (972.6935, 738.3949)
  point P23 (663.4235, 0)
  point P24 (663.4235, 0)
  point P25 (854.1183, 777.5027)
  point P26 (663.4235, 0)
  point P27 (663.4235, 0)
  point P28 (730.9044, 797.6974)
  point P29 (663.4235, 0)
  point P30 (663.4235, 0)
  point P31 (606.0491, 798.488)
  point P32 (663.4235, 0)
  point P33 (663.4235, 0)
  point P34 (482.5894, 779.855)
  point P35 (663.4235, 0)
  point P36 (663.4235, 0)
  point P37 (363.5285, 742.2519)
  point P38 (663.4235, 0)
  point P39 (663.4235, 0)
  point P40 (251.7627, 686.5932)
  point P41 (663.4235, 0)
  point P42 (663.4235, 0)
  point P43 (150.0106, 614.2329)
  point P44 (663.4235, 0)
  point P45 (663.4235, 0)
  point P46 (60.7475, 526.9312)
  point P47 (663.4235, 0)
  point P48 (663.4235, 0)
  point P49 (-13.8553, 426.8117)
  point P50 (663.4235, 0)
  point P51 (663.4235, 0)
  point P52 (-71.9831, 316.3099)
  point P53 (663.4235, 0)
  point P54 (663.4235, 0)
  point P55 (-112.2219, 198.1137)
  point P56 (663.4235, 0)
  point P57 (663.4235, 0)
  point P58 (-133.5928, 75.0984)
  point P59 (663.4235, 0)
  dimension "d92" = 10
  dimension "d93" = 65
  dimension "d94" = 5.015
  dimension "d97" = 169.96
  constraints: 160 end point, 21 coincident, 20 point on line, 2 parallel, 1 midpoint, 1 perpendicular, 1 point on circle, 247 other
  measures "d92" distance between parallel lines of L0 L2
  measures "d93" distance from line of L4 point (1461.327, 65)
  measures "d94" angle of L4 L0
extrude "Extrusion5" cut sketch "Sketch7" against normal up to surface (830 mm away) contours L3 L8 L5 L2 A1 L0 | A1 L2 L1 L0 | L8 L7 L77 L2 L3 | L12 L11 L77 L7 L8 | L12 L9 L2 L5 L8 | L16 L15 L77 L11 L12 | L16 L13 L2 L9 L12 | L20 L19 L77 L15 L16 | L20 L17 L2 L13 L16 | L24 L23 L77 L19 L20 | L24 L21 L2 L17 L20 | L28 L27 L77 L23 L24 | L28 L25 L2 L21 L24 | L32 L31 L77 L27 L28 | L32 L29 L2 L25 L28 | L36 L35 L77 L31 L32 | L36 L33 L2 L29 L32 | L40 L39 L77 L35 L36 | L40 L37 L2 L33 L36 | L44 L43 L77 L39 L40 | L44 L41 L2 L37 L40 | L48 L47 L77 L43 L44 | L48 L45 L2 L41 L44 | L52 L51 L77 L47 L48 | L52 L49 L2 L45 L48 | L56 L55 L77 L51 L52 | L56 L53 L2 L49 L52 | L60 L59 L77 L55 L56 | L60 L57 L2 L53 L56 | L64 L63 L77 L59 L60 | L64 L61 L2 L57 L60 | L68 L67 L77 L63 L64 | L68 L65 L2 L61 L64 | L72 L71 L77 L67 L68 | L72 L69 L2 L65 L68 | L76 L75 L77 L71 L72 | L76 L73 L2 L69 L72 | L80 L79 L78 L77 L75 L76 | L80 L77 L2 L73 L76 | L3 L2 L77 L80 | L2 L9 L7 A1 L5 | A1 L7 L6 L5 | L77 L7 L73 L2 | L77 L11 L73 L7 | L77 L15 L73 L11 | L2 L13 L7 L9 | L77 L19 L73 L15 | L2 L17 L7 L13 | L77 L23 L73 L19 | L2 L21 L7 L17 | L77 L27 L73 L23 | L2 L25 L7 L21 | L77 L31 L73 L27 | L2 L29 L7 L25 | L77 L35 L73 L31 | L2 L33 L7 L29 | L77 L39 L73 L35 | L2 L37 L7 L33 | L77 L43 L73 L39 | L2 L41 L7 L37 | L77 L47 L73 L43 | L2 L45 L7 L41 | L77 L51 L73 L47 | L2 L49 L7 L45 | L77 L55 L73 L51 | L2 L53 L7 L49 | L77 L59 L73 L55 | L2 L57 L7 L53 | L77 L63 L73 L59 | L2 L61 L7 L57 | L77 L67 L73 L63 | L2 L65 L7 L61 | L77 L71 L73 L67 | L2 L69 L7 L65 | L77 L75 L74 L73 L71 | L2 L73 L7 L69 | L73 L11 L69 L7 | L73 L15 L69 L11 | L7 L13 L11 A1 L9 | L73 L19 L69 L15 | L7 L17 L11 L13 | L73 L23 L69 L19 | L7 L21 L11 L17 | L73 L27 L69 L23 | L7 L25 L11 L21 | L73 L31 L69 L27 | L7 L29 L11 L25 | L73 L35 L69 L31 | L7 L33 L11 L29 | L73 L39 L69 L35 | L7 L37 L11 L33 | L73 L43 L69 L39 | L7 L41 L11 L37 | L73 L47 L69 L43 | L7 L45 L11 L41 | L73 L51 L69 L47 | L7 L49 L11 L45 | L73 L55 L69 L51 | L7 L53 L11 L49 | L73 L59 L69 L55 | L7 L57 L11 L53 | L73 L63 L69 L59 | L7 L61 L11 L57 | L73 L67 L69 L63 | L7 L65 L11 L61 | L73 L71 L70 L69 L67 | L7 L69 L11 L65 | A1 L11 L10 L9 | L69 L15 L65 L11 | L69 L19 L65 L15 | L11 L17 L15 A1 L13 | L69 L23 L65 L19 | L11 L21 L15 L17 | L69 L27 L65 L23 | L11 L25 L15 L21 | L69 L31 L65 L27 | L11 L29 L15 L25 | L69 L35 L65 L31 | L11 L33 L15 L29 | L69 L39 L65 L35 | L11 L37 L15 L33 | L69 L43 L65 L39 | L11 L41 L15 L37 | L69 L47 L65 L43 | L11 L45 L15 L41 | L69 L51 L65 L47 | L11 L49 L15 L45 | L69 L55 L65 L51 | L11 L53 L15 L49 | L69 L59 L65 L55 | L11 L57 L15 L53 | L69 L63 L65 L59 | L11 L61 L15 L57 | L69 L67 L66 L65 L63 | L11 L65 L15 L61 | L65 L19 L61 L15 | A1 L15 L14 L13 | L65 L23 L61 L19 | L15 L21 L19 A1 L17 | L65 L27 L61 L23 | L15 L25 L19 L21 | L65 L31 L61 L27 | L15 L29 L19 L25 | L65 L35 L61 L31 | L15 L33 L19 L29 | L65 L39 L61 L35 | L15 L37 L19 L33 | L65 L43 L61 L39 | L15 L41 L19 L37 | L65 L47 L61 L43 | L15 L45 L19 L41 | L65 L51 L61 L47 | L15 L49 L19 L45 | L65 L55 L61 L51 | L15 L53 L19 L49 | L65 L59 L61 L55 | L15 L57 L19 L53 | L65 L63 L62 L61 L59 | L15 L61 L19 L57 | L61 L23 L57 L19 | A1 L19 L18 L17 | L61 L27 L57 L23 | L19 L25 L23 L22 L21 | L61 L31 L57 L27 | L19 L29 L23 L25 | L61 L35 L57 L31 | L19 L33 L23 L29 | L61 L39 L57 L35 | L19 L37 L23 L33 | L61 L43 L57 L39 | L19 L41 L23 L37 | L61 L47 L57 L43 | L19 L45 L23 L41 | L61 L51 L57 L47 | L19 L49 L23 L45 | L61 L55 L57 L51 | L19 L53 L23 L49 | L61 L59 L58 L57 L55 | L19 L57 L23 L53 | L57 L27 L53 L23 | L57 L31 L53 L27 | L23 L29 L27 L26 L25 | L57 L35 L53 L31 | L23 L33 L27 L29 | L57 L39 L53 L35 | L23 L37 L27 L33 | L57 L43 L53 L39 | L23 L41 L27 L37 | L57 L47 L53 L43 | L23 L45 L27 L41 | L57 L51 L53 L47 | L23 L49 L27 L45 | L57 L55 L54 L53 L51 | L23 L53 L27 L49 | L53 L31 L49 L27 | L53 L35 L49 L31 | L27 L33 L31 L30 L29 | L53 L39 L49 L35 | L27 L37 L31 L33 | L53 L43 L49 L39 | L27 L41 L31 L37 | L53 L47 L49 L43 | L27 L45 L31 L41 | L53 L51 L50 L49 L47 | L27 L49 L31 L45 | L49 L35 L45 L31 | L49 L39 L45 L35 | L31 L37 L35 L34 L33 | L49 L43 L45 L39 | L31 L41 L35 L37 | L49 L47 L46 L45 L43 | L31 L45 L35 L41 | L45 L39 L41 L35 | L45 L43 L42 L41 L39 | L35 L41 L39 L38 L37 bodies 2
sketch "Sketch8" plane through (275, 370.625, -490.5099) normal (0, 1, 0) x (1, 0, 0)
  line L0 (240, 0) -> (0, 0)
  line L1 (0, 0) -> (0, 380)
  line L2 (0, 380) -> (240, 380)
  line L3 (240, 380) -> (240, 0)
  line L4 (-550, 0) -> (-790, 0)
  line L5 (-790, 0) -> (-790, 380)
  line L6 (-790, 380) -> (-550, 380)
  line L7 (-550, 380) -> (-550, 0)
  point P0 (-275, -490.5099)
  point P1 (0, 380)
  constraints: 16 end point, 4 coincident, 4 parallel, 2 horizontal, 2 perpendicular
extrude "Extrusion6" cut sketch "Sketch8" against normal up to surface (830 mm away) bodies 1 2
sketch "Sketch9" plane through (0, -519.375, 0) normal (0, -1, 0) x (1, 0, 0)
  line L0 (515, -870.5099) -> (-515, -870.5099)
  line L1 (-515, -870.5099) -> (-515, -373.9082)
  line L2 (-515, -373.9082) -> (515, -373.9082)
  line L3 (515, -373.9082) -> (515, -870.5099)
  arc A0 (-636.4215, 0) -> (636.4215, 0) centre (0, 0) ccw projected
  point P0 (0, 0)
  point P1 (-515, -490.5099)
  constraints: 8 end point, 2 parallel, 1 coincident, 1 horizontal, 1 perpendicular, 1 point on circle, 1 point on line
extrude "Extrusion7" add sketch "Sketch9" against normal up to surface (60 mm away) bodies 2
sketch "Sketch10" plane through (0, 0, 0) normal (0, 0, 1) x (1, 0, 0)
  circle A0 centre (0, 0) radius 562.717 construction
  circle A1 centre (0, 494.7917) radius 354.1667 construction
  line L0 (636.4215, -459.375) -> (-636.4215, -459.375) construction
  arc A2 (-350, 440.625) -> (350, 440.625) centre (0, 494.7917) ccw
  arc A3 (-350, 440.625) -> (-325, -459.375) centre (0, 0) ccw
  arc A4 (325, -459.375) -> (350, 440.625) centre (0, 0) ccw
  line L1 (325, -459.375) -> (-325, -459.375)
  line L2 (-350, 440.625) -> (350, 440.625)
  dimension "d105" = 600
  dimension "d106" = 300
  dimension "d107" = 650
  dimension "d108" = 700
  constraints: 12 point on circle, 4 end point, 3 centre point, 3 concentric, 2 point on line, 1 horizontal
  measures "d105" distance edge to line of A1 L0
  measures "d106" distance edge to line of A1 L2
  measures "d107" distance of L1.start L1.end
  measures "d108" distance of L2.start L2.end
body "Solid1"
body "Solid2"
body "Solid3"
